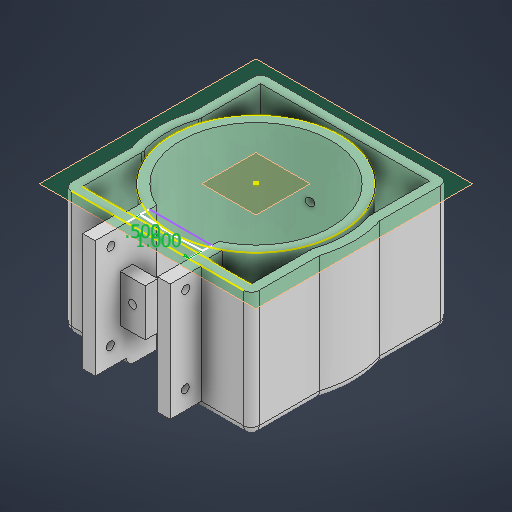
# Autodesk Inventor part: I-bolt compatable floater for in-situ water detection v5
Saved by Autodesk Inventor 2026 (Build 300175050, 175E)
## iProperties
Created: 2025-05-30
Part Number: I-bolt compatable floater for in-situ water detection v5
Material: Generic
Document SubType Name: Modeling
Designer: localuser
Density: 1 g/cm^3
Appearance: Default
Author: localuser
Autodesk Inventor part; units mm, degrees
ref_plane "YZ Plane" through (0, 0, 0) normal (1, 0, 0) x (0, 1, 0)
ref_plane "XZ Plane" through (0, 0, 0) normal (0, 1, 0) x (-1, 0, 0)
ref_plane "XY Plane" through (0, 0, 0) normal (0, 0, 1) x (1, 0, 0)
sketch "Sketch1" plane through (0, 0, 0) normal (0, 1, 0) x (-1, 0, 0)
  circle A0 centre (0, 0) radius 40.005
  dimension "d0" = 80.01
  constraints: 1 centre point, 1 coincident
  measures "d0" diameter of A0
extrude "Extrusion1" add sketch "Sketch1" along normal blind 50.8
ref_plane "Work Plane2" through (0, 50.8, 0) normal (0, 1, 0) x (1, 0, 0)
sketch "Sketch2" plane through (0, 50.8, 0) normal (0, 1, 0) x (1, 0, 0)
  circle A0 centre (0, 0) radius 30.48
  dimension "d5" = 60.96
  constraints: 1 centre point, 1 coincident
  measures "d5" diameter of A0
hole "Hole1" at (0, 50.8, 0) direction (0, -1, 0) diameter 60.96 end through all
ref_plane "Work Plane1" through (0, 50.8, 0) normal (0, 1, 0) x (1, 0, 0)
sketch "Sketch3" plane through (0, 50.8, 0) normal (0, 1, 0) x (1, 0, 0)
  line L0 (0, -31.4608) -> (0, -36.83)
  circle A0 centre (0, 0) radius 36.83 projected
  circle A1 centre (0, 0) radius 30.48 projected
  line L1 (0, -30.48) -> (38.1, -30.48)
  line L2 (38.1, -30.48) -> (38.1, -40.005)
  line L3 (38.1, -40.005) -> (0, -40.005)
  line L4 (0, -40.005) -> (0, -30.48)
  line L5 (0, -40.005) -> (0, -30.48)
  line L6 (0, -30.48) -> (-38.1, -30.48)
  line L7 (-38.1, -30.48) -> (-38.1, -40.005)
  line L8 (-38.1, -40.005) -> (0, -40.005)
  circle A2 centre (0, 0) radius 40.005 projected
  arc A3 (0, -40.005) -> (25.9108, -30.48) centre (0, 0) ccw
  arc A4 (0, -40.005) -> (-25.9108, -30.48) centre (0, 0) ccw
  dimension "d13" = 38.1
  dimension "d14" = 38.1
  constraints: 18 end point, 7 point on circle, 4 parallel, 2 centre point, 2 perpendicular, 2 point on line, 2 vertical alignment, 1 horizontal, 1 tangent, 1 vertical, 2 other
  measures "d13" distance of L2.end L3.end
  measures "d14" distance of L6.end L1.start
extrude "Extrusion2" add sketch "Sketch3" against normal blind 50.8 contours A2 L1 L2 L3 | L8 L7 L6 A2
ref_plane "Work Plane3" through (38.1, 50.8, 40.005) normal (0, -1, 0) x (0, 0, -1)
sketch "Sketch4" plane through (0, 50.8, 0) normal (0, 1, 0) x (1, 0, 0)
  line L0 (-38.1, -40.005) -> (-38.1, -30.48) projected
  line L1 (38.1, 40.005) -> (-38.1, 40.005)
  line L2 (-38.1, 40.005) -> (-38.1, -40.005)
  line L3 (-38.1, -40.005) -> (38.1, -40.005)
  line L4 (38.1, -40.005) -> (38.1, 40.005)
  line L5 (38.1, 40.005) -> (-38.1, -40.005) construction
  line L6 (-38.1, 40.005) -> (38.1, -40.005) construction
  arc A0 (25.9108, -30.48) -> (-25.9108, -30.48) centre (0, 0) ccw projected
  arc A1 (-25.9108, -30.48) -> (-38.1, -12.198) centre (0, 0) ccw
  line L7 (-38.1, -30.48) -> (-25.9108, -30.48) projected
  line L8 (-25.9108, -30.48) -> (-38.1, -30.48)
  line L9 (-38.1, -30.48) -> (-38.1, -12.198)
  line L10 (25.9108, -30.48) -> (38.1, -30.48)
  point P0 (38.1, -12.198)
  point P1 (0, 40.005)
  point P2 (38.1, 12.198)
  point P3 (-38.1, 12.198)
  constraints: 18 end point, 3 equal length, 3 point on circle, 3 point on line, 2 midpoint, 1 centre point, 1 horizontal, 1 perpendicular
extrude "Extrusion3" add sketch "Sketch4" against normal blind 50.8 contours L2 A0 L7 | A0 L4 L10 | L2 L1 A0 | L1 L4 A0
shell "Shell1" thickness 3.81 removed faces 1 at (0, 50.8, -36.83)
fillet "Fillet3" radius 3.175 8 edges at (38.1, 0, -26.1015) (40.005, 0, 0) (38.1, 0, 26.1015) (0, 0, 40.005) (0, 0, -40.005) (-38.1, 0, -26.1015) (-40.005, 0, 0) (-38.1, 0, 26.1015)
fillet "Fillet4" radius 3.175 8 edges at (-37.1701, 0.9299, 39.0751) (-38.1, 26.9875, 40.005) (-37.1701, 0.9299, -39.0751) (-38.1, 26.9875, -40.005) (37.1701, 0.9299, -39.0751) (38.1, 26.9875, -40.005) (37.1701, 0.9299, 39.0751) (38.1, 26.9875, 40.005)
sketch "Sketch6" plane through (0, 50.8, 0) normal (0, 1, 0) x (1, 0, 0)
  point P0 (0, 0)
sketch "Sketch7" plane through (34.925, 50.8, -40.005) normal (0, 0, -1) x (-1, 0, 0)
  line L0 (-5.08, -47.625) -> (-3.175, -47.625) projected
  line L1 (-3.175, -47.625) -> (34.925, -46.99)
  line L2 (0.635, -46.99) -> (69.215, -46.99) projected
  line L3 (69.85, 0) -> (0, 0) projected
  line L4 (34.925, 0) -> (34.925, -26.7586)
  line L5 (34.925, 0) -> (34.925, -25.4)
  line L6 (9.525, -10.8332) -> (60.325, -10.8332)
  line L7 (60.325, -10.8332) -> (60.325, -39.9668)
  line L8 (60.325, -39.9668) -> (9.525, -39.9668)
  line L9 (9.525, -39.9668) -> (9.525, -10.8332)
  line L10 (9.525, -10.8332) -> (60.325, -39.9668) construction
  line L11 (60.325, -10.8332) -> (9.525, -39.9668) construction
  point P0 (34.925, -50.8)
  dimension "d23" = 25.4
  dimension "d24" = 50.8
  constraints: 18 end point, 4 midpoint, 2 parallel, 1 horizontal, 1 perpendicular, 1 point on line, 1 vertical
  measures "d23" distance of L4.start L5.end
  measures "d24" distance of L7.end L8.end
extrude "Extrusion4" add sketch "Sketch7" along normal blind 12.7
sketch "Sketch8" plane through (-25.4, 39.9668, -40.005) normal (0, 1, 0) x (1, 0, 0)
  line L0 (0, 12.7) -> (50.8, 12.7) projected
  line L1 (50.8, 12.7) -> (25.4, 12.7)
  circle A0 centre (25.4, 6.3494) radius 4.0427
  point P0 (25.4, -40.005)
  constraints: 2 end point, 1 centre point, 1 midpoint
hole "Hole2" at (0, 39.9668, -46.3544) direction (0, -1, 0) diameter 5.1054 end through all
fillet "Fillet5" radius 3.175 8 edges at (0, 10.8332, -52.705) (25.4, 10.8332, -46.355) (-25.4, 10.8332, -46.355) (25.4, 25.4, -52.705) (-25.4, 25.4, -52.705) (0, 39.9668, -52.705) (25.4, 39.9668, -46.355) (-25.4, 39.9668, -46.355)
sketch "Sketch9" plane through (0, 50.8, 0) normal (0, 1, 0) x (1, 0, 0)
  circle A0 centre (0, 0) radius 34.29 projected
  line L0 (0, -34.29) -> (-12.7, -34.29)
  line L1 (-12.7, -34.29) -> (12.7, -34.29)
  line L2 (-12.7, -34.29) -> (-12.7, -30.6147)
  line L3 (34.29, -36.195) -> (-34.29, -36.195) projected
  line L4 (-12.7, -30.6147) -> (12.7, -30.6147)
  line L5 (12.7, -30.6147) -> (12.7, -34.29)
  line L6 (-12.7, -34.29) -> (-12.7, -40.005)
  line L7 (34.925, -40.005) -> (-34.925, -40.005) projected
  line L8 (12.7, -40.005) -> (12.7, -30.6147)
  dimension "d35" = 12.7
  dimension "d36" = 25.4
  constraints: 14 end point, 5 perpendicular, 3 point on line, 2 horizontal, 1 vertical alignment, 1 other
  measures "d35" distance of L0.start L0.end
  measures "d36" distance of L0.end L1.end
sketch "Sketch10" plane through (0, 50.8, 0) normal (0, 1, 0) x (1, 0, 0)
  line L0 (34.925, -40.005) -> (-34.925, -40.005) projected
  line L1 (34.29, -36.195) -> (-34.29, -36.195) projected
  line L2 (12.7297, -40.005) -> (-12.6433, -40.005)
  line L3 (-12.6433, -40.005) -> (-12.6433, -36.195)
  line L4 (-12.6433, -36.195) -> (12.7297, -36.195)
  line L5 (12.7297, -36.195) -> (12.7297, -40.005)
  point P0 (0, 0)
  constraints: 8 end point, 2 parallel, 2 point on line, 1 horizontal, 1 perpendicular
extrude "Extrusion5" cut sketch "Sketch10" against normal blind 50.8
sketch "Sketch12" plane through (0, 50.8, 0) normal (0, 1, 0) x (1, 0, 0)
  line L0 (12.7297, -36.195) -> (12.7297, -40.005) projected
  line L1 (12.7297, -36.195) -> (12.7297, -27.6945)
  circle A0 centre (0, 0) radius 30.48 projected
  line L2 (-12.6433, -36.195) -> (-34.29, -36.195) projected
  line L3 (-12.6433, -27.6945) -> (-12.6433, -36.195)
  line L4 (-12.6433, -36.195) -> (12.7297, -36.195)
  line L5 (12.7297, -27.6945) -> (-12.6433, -27.6945)
  point P0 (-12.6433, -27.734)
  constraints: 8 end point, 2 vertical, 1 parallel, 1 perpendicular, 2 other
extrude "Extrusion6" cut sketch "Sketch12" against normal blind 50.8 contours L4 L3 A0 L1
sketch "Sketch13" plane through (0, 50.8, 0) normal (0, 1, 0) x (1, 0, 0)
  line L0 (12.7297, -40.005) -> (34.925, -40.005) projected
  line L1 (12.7297, -27.6945) -> (12.7297, -31.8396) projected
  line L2 (12.7297, -40.005) -> (12.7297, -27.6945)
  line L3 (12.7297, -27.6945) -> (16.5325, -27.6945)
  line L4 (16.5325, -27.6945) -> (16.5325, -40.005)
  line L5 (16.5325, -40.005) -> (12.7297, -40.005)
  line L6 (-12.6433, -40.005) -> (-12.6433, -27.6945)
  line L7 (-12.6433, -27.6945) -> (-16.4533, -27.6945)
  line L8 (-16.4533, -27.6945) -> (-16.4533, -40.005)
  line L9 (-16.4533, -40.005) -> (-12.6433, -40.005)
  line L10 (34.29, -36.195) -> (12.7297, -36.195) projected
  line L11 (16.5325, -36.195) -> (12.7297, -36.195)
  line L12 (12.7297, -36.195) -> (12.7297, -31.8396)
  line L13 (12.7297, -36.195) -> (16.5325, -36.195)
  line L14 (16.5325, -30.0795) -> (16.5325, -36.195)
  arc A0 (12.7297, -31.8396) -> (16.5325, -30.0795) centre (-4.777, 10.9733) ccw
  arc A1 (12.7297, -31.8396) -> (-12.6433, -31.874) centre (0, 0) ccw projected
  arc A2 (-16.4533, -30.0847) -> (-12.6433, -31.874) centre (0, 0) ccw
  line L15 (-16.4533, -30.0847) -> (-16.4533, -36.195)
  line L16 (-12.6433, -36.195) -> (-34.29, -36.195) projected
  line L17 (-12.6433, -36.195) -> (-12.6433, -31.874)
  point P0 (14.6311, -31.0119)
  dimension "d41" = 3.81
  constraints: 28 end point, 6 point on line, 5 collinear, 5 point on circle, 4 parallel, 3 perpendicular, 2 centre point, 1 vertical
  measures "d41" distance of L7.end L6.end
extrude "Extrusion7" add sketch "Sketch13" against normal blind 50.8 contours L2 A1 A0 L4 L10 | L16 L8 A1 L6
sketch "Sketch14" plane through (34.925, 3.175, 40.005) normal (0, 0, 1) x (1, 0, 0)
  line L0 (-22.1953, 47.625) -> (-22.1953, 0) projected
  line L1 (-22.1953, 47.625) -> (-22.1953, 22.225)
  line L2 (-22.1953, 22.225) -> (-47.5683, 22.225)
  line L3 (-47.5683, 0) -> (-47.5683, 47.625) projected
  line L4 (-22.1953, 47.625) -> (-22.1953, 0)
  line L5 (-22.1953, 0) -> (-17.1153, 0)
  line L6 (-17.1153, 0) -> (-17.1153, 47.625)
  line L7 (-17.1153, 47.625) -> (-22.1953, 47.625)
  line L8 (-47.5683, 0) -> (-47.5683, 47.625)
  line L9 (-47.5683, 47.625) -> (-52.6483, 47.625)
  line L10 (-52.6483, 47.625) -> (-52.6483, 0)
  line L11 (-52.6483, 0) -> (-47.5683, 0)
  point P0 (-34.925, -3.175)
  dimension "d44" = 25.4
  dimension "d45" = 5.08
  dimension "d46" = 5.08
  constraints: 20 end point, 6 equal length, 3 perpendicular, 2 point on line
  measures "d44" distance of L0.start L1.end
  measures "d45" distance of L5.end L0.end
  measures "d46" distance of L9.end L3.end
extrude "Extrusion8" add sketch "Sketch14" along normal blind 12.7
sketch "Sketch15" plane through (17.8097, 3.175, 40.005) normal (1, 0, 0) x (0, 0, -1)
  line L0 (-12.7, 47.625) -> (-12.7, 0) projected
  line L1 (-12.7, 47.625) -> (-6.35, 47.625)
  line L2 (12.271, 47.625) -> (-12.7, 47.625) projected
  line L3 (-6.35, 47.625) -> (-6.35, 42.545)
  line L4 (-6.35, 42.545) -> (-6.35, 45.085)
  line L5 (-12.7, 0) -> (-5.6902, 0)
  line L6 (-5.6902, 0) -> (-0.2145, 0)
  line L7 (-0.2145, 0) -> (-6.5645, 0)
  line L8 (-6.5645, 0) -> (-6.5645, 7.62)
  point P0 (40.005, -3.175)
  dimension "d49" = 6.35
  dimension "d50" = 5.08
  dimension "d51" = 2.54
  dimension "d52" = 6.35
  dimension "d53" = 7.62
  constraints: 14 end point, 3 point on line, 2 perpendicular, 1 horizontal, 1 midpoint
  measures "d49" distance of L0.start L1.end
  measures "d50" distance of L1.end L3.end
  measures "d51" distance of L3.end L4.end
  measures "d52" distance of L6.end L7.end
  measures "d53" distance of L7.end L8.end
hole "Hole3" at (17.8097, 45.72, 46.355) at (17.8097, 10.795, 46.5695) direction (-1, 0, 0) diameter 3.175 end through all
sketch "Sketch16" plane through (-12.6433, 0, 27.734) normal (1, 0, 0) x (0, 0, -1)
  line L0 (-24.971, 3.175) -> (-24.971, 50.8) projected
  line L1 (-24.971, 50.8) -> (-24.971, 25.4)
  line L2 (-24.971, 25.4) -> (-12.271, 25.4)
  line L3 (-14.811, 15.8805) -> (-9.731, 15.8805)
  line L4 (-9.731, 15.8805) -> (-9.731, 34.9195)
  line L5 (-9.731, 34.9195) -> (-14.811, 34.9195)
  line L6 (-14.811, 34.9195) -> (-14.811, 15.8805)
  line L7 (-14.811, 15.8805) -> (-9.731, 34.9195) construction
  line L8 (-9.731, 15.8805) -> (-14.811, 34.9195) construction
  point P0 (27.734, 0)
  dimension "d61" = 25.4
  dimension "d62" = 12.7
  dimension "d63" = 5.08
  constraints: 16 end point, 2 midpoint, 2 parallel, 2 perpendicular, 1 horizontal, 1 point on line
  measures "d61" distance of L0.end L1.end
  measures "d62" distance of L1.end L2.end
  measures "d63" distance of L5.end L4.end
extrude "Extrusion9" add sketch "Sketch16" along normal blind 10.16
sketch "Sketch17" plane through (-12.6433, 15.8805, 42.545) normal (0, 0, 1) x (1, 0, 0)
  line L0 (0, 19.039) -> (10.16, 19.039) projected
  line L1 (10.16, 19.039) -> (5.08, 19.039)
  line L2 (5.08, 10.0369) -> (5.08, 19.039)
  point P0 (12.6433, -15.8805)
  constraints: 4 end point, 1 midpoint, 1 perpendicular
hole "Hole4" at (-7.5633, 25.9174, 42.545) direction (0, 0, -1) diameter 3.175 end through all
body "Solid1"
